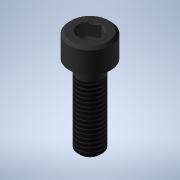
# Autodesk Inventor part: DIN-912 - M5x16(F)
Saved by Autodesk Inventor 2021 (Build 250183000, 183)
## iProperties
Created: 2026-04-18
Part Number: DIN-912 - M5x16(F)
Material: Generic
Catalog Web Link: www.3dfindit.com
Description: DIN-912-Cylinder screw
Vendor: FESTO
Document SubType Name: Modeling
Designer: psAdmin
Manufacturer: FESTO
Mass: 0.55311 g
Surface Area: 5.1769 cm^2
Volume: 0.55311 cm^3
Density: 1 g/cm^3
Appearance: PSOLRGB-176-176-176
Category: PARTsolutions
Company: FESTO
Title: DIN-912 - M5x16(F)
Author: Cadenas PARTsolutions
Comments: Cylinder screw
PSOL_IDENT_0: {$CADENAS_DATA/23d-libs/festo/zyl_zubeh/d912/din_912.prj},178 {VTYP=3D},{NB=DIN-912 - M5x16(F)},{LIN
PSOL_IDENT_1: A=DIN-912 - M5x16(F)},{NN=DIN-912},{DATE=25.11.2021 14:13:45},{GEOMDATE=25.11.2021 14:12:35},{VERSIO
PSOL_IDENT_2: N=},{LINEID=340},{WBVAR=},{WBNUMERIC=}  {NB=DIN-912 - M5x16(F)},{LINA=DIN-912 - M5x16(F)},{KT=X},{ID
PSOL_IDENT_3: NR=},{GEW=M5},{DG=5.000},{P=0.800},{L=16.000},{B=16.000},{FORM=1},{GKD=4.019},{DK=8.500},{DADIN=5.70
PSOL_IDENT_4: 0},{DS=5.000},{E=4.580},{LF=0.600},{K=5.000},{R=0.200},{S=4.000},{T=2.500},{V=0.500},{DW=8.030},{W=1
PSOL_IDENT_5: .900},{NENN=M5x16},{DA=5.1},{BL=13.6}
NB: DIN-912 - M5x16(F)
NN: DIN-912
NT: Cylinder screw
NBSYN: DIN-912 - $NENN.(F)
LINA: DIN-912 - M5x16(F)
CATALOG: Festo
ROWDESC: M5x16
GEW: M5
DG: 5
P: 0.8
L: 16
B: 16
FORM: 1
GKD: 4.019
DK: 8.5
DADIN: 5.7
DS: 5
E: 4.58
LF: 0.6
K: 5
R: 0.2
S: 4
T: 2.5
V: 0.5
DW: 8.03
W: 1.9
SUPPLIER: FESTO
ARTICLENO: DIN-912 - M5x16(F)
BOMINFO: DIN-912 - M5x16(F)
CREATOR: CADENAS GmbH
Autodesk Inventor part; units mm, degrees
sketch "Sketch_1" plane through (0, 0, 0) normal (0, 0, 1) x (1, 0, 0)
  line L0 (0, -16) -> (0, 5)
  line L1 (0, 1.3453) -> (2, 2.5)
  line L2 (2, 2.5) -> (2, 4.6906)
  line L3 (2, 4.6906) -> (2.3094, 5)
  line L4 (2.3094, 5) -> (3.75, 5)
  line L5 (3.75, 5) -> (4.25, 4.5)
  line L6 (4.25, 4.5) -> (4.25, 0.125)
  line L7 (4.25, 0.125) -> (4.125, 0)
  line L8 (4.125, 0) -> (2.55, 0)
  line L9 (2.55, 0) -> (2.5, -0.6)
  line L10 (2.5, -0.6) -> (2.5, -15.5095)
  line L11 (2.5, -15.5095) -> (2.0095, -16)
  line L12 (2.0095, -16) -> (0, -16)
  line L13 (0, -16) -> (0, 1.3453)
  constraints: 28 end point
revolve "Revolution1" add sketch "Sketch_1" angle 360 about axis through (0, -16, 0) along (0, -1, 0)
thread "Thread1" size "M5x0.8" class "6g" standard "ISO Metric profile" length 13.1095
sketch "Sketch_2" plane through (0, 5, 0) normal (0, 1, 0) x (1, 0, 0)
  line L0 (-2, -1.1547) -> (0, -2.3094)
  line L1 (0, -2.3094) -> (2, -1.1547)
  line L2 (2, -1.1547) -> (2, 1.1547)
  line L3 (2, 1.1547) -> (0, 2.3094)
  line L4 (0, 2.3094) -> (-2, 1.1547)
  line L5 (-2, 1.1547) -> (-2, -1.1547)
  constraints: 12 end point
extrude "Extrusion1" cut sketch "Sketch_2" against normal blind 2.5
ref_plane "ANBAU_XY" through (0, 0, 0) normal (0, 1, 0) x (1, 0, 0)
ref_plane "ANBAU_YZ" through (0, 0, 0) normal (1, 0, 0) x (0, 0, -1)
ref_plane "ANBAU_ZX" through (0, 0, 0) normal (0, 0, -1) x (0, 1, 0)
ref_plane "Schraube_XY" through (0, 0, 0) normal (0, 1, 0) x (1, 0, 0)
ref_plane "Schraube_YZ" through (0, 0, 0) normal (1, 0, 0) x (0, 0, -1)
ref_plane "Schraube_ZX" through (0, 0, 0) normal (0, 0, -1) x (0, 1, 0)
ref_plane "insert_XY" through (0, 0, 0) normal (0, 1, 0) x (1, 0, 0)
ref_plane "insert_YZ" through (0, 0, 0) normal (1, 0, 0) x (0, 0, -1)
ref_plane "insert_ZX" through (0, 0, 0) normal (0, 0, -1) x (0, 1, 0)
ref_plane "schrauben_punkt_XY" through (0, -16, 0) normal (0, 1, 0) x (1, 0, 0)
ref_plane "schrauben_punkt_YZ" through (0, -16, 0) normal (1, 0, 0) x (0, 0, -1)
ref_plane "schrauben_punkt_ZX" through (0, -16, 0) normal (0, 0, -1) x (0, 1, 0)
body "Solid1"
